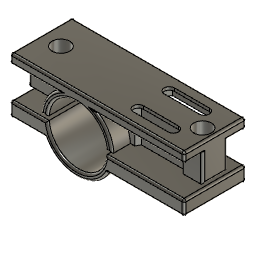
plate_holder (Autodesk Fusion 360 design; units mm, degrees)
Autodesk Fusion 360 part; units mm, degrees
sketch "Sketch1" plane through (0, 0, 0) normal (0, 1, 0) x (1, 0, 0)
  line L0 (17.1709, 1) -> (52.1709, 1)
  line L1 (52.1709, 1) -> (52.1709, 8)
  line L2 (52.1709, 8) -> (15.2263, 8)
  line L3 (17.1709, 1) -> (14.1647, 1)
  line L4 (0, 0) -> (0, 14.2)
  line L5 (-32.1709, 8) -> (-15.2263, 8)
  line L6 (-32.1709, 1) -> (-32.1709, 8)
  line L7 (-17.1709, 1) -> (-32.1709, 1)
  line L8 (-17.1709, 1) -> (-14.1647, 1)
  arc A0 (17.1709, 1) -> (-17.1709, 1) centre (0, 0) ccw
  arc A1 (14.1647, 1) -> (-14.1647, 1) centre (0, 0) ccw
  dimension "d1" = 28.4
  dimension "d3" = 1
  dimension "d4" = 7
  dimension "d5" = 35
  dimension "d6" = 34.4
  dimension "d64" = 15
  dimension "d65" = 7
  dimension "d66" = 1
  constraint coincident L4.start A0.centre
  constraint horizontal L0
  constraint perpendicular L0 L1
  constraint perpendicular L1 L2
  constraint parallel L0 L3
  constraint coincident L4.end A1
  constraint vertical L4
  constraint concentric A0 A1
  constraint coincident L5.end A0
  constraint parallel L0 L7
  constraint parallel L1 L6
  constraint parallel L2 L5
  constraint parallel L3 L8
  measures "d1" diameter of A1
  measures "d3" distance of L4.start L0
  measures "d4" distance of L0.end L1.end
  measures "d5" horizontal distance of L0.start L1.end
  measures "d6" diameter of A0
  measures "d64" distance of L6.start L7.start
  measures "d65" distance of L5.start L6.start
  measures "d66" distance of L7 L4.start
extrude "Extrude1" add sketch "Sketch1" along normal blind 30 makes body 1
sketch "Sketch2" plane through (0, 0, 0) normal (0, 1, 0) x (1, 0, 0)
  line L0 (17.1709, -1) -> (52.1709, -1)
  line L1 (52.1709, -1) -> (52.1709, -19)
  line L2 (52.1709, -19) -> (0, -19)
  line L3 (17.1709, -1) -> (14.1647, -1)
  line L4 (0, 0) -> (0, -19)
  line L5 (-32.1709, -19) -> (0, -19)
  line L6 (-32.1709, -1) -> (-32.1709, -19)
  line L7 (-17.1709, -1) -> (-32.1709, -1)
  line L8 (-17.1709, -1) -> (-14.1647, -1)
  arc A0 (-17.1709, -1) -> (17.1709, -1) centre (0, 0) ccw
  arc A1 (-14.1647, -1) -> (14.1647, -1) centre (0, 0) ccw
  line L9 (0, -14.2) -> (52.1709, -14.2)
  line L10 (0, -14.2) -> (-32.1709, -14.2)
  dimension "d9" = 28.4
  dimension "d10" = 34.4
  dimension "d11" = 1
  dimension "d12" = 35
  dimension "d14" = 18
  dimension "d67" = 18
  dimension "d68" = 15
  dimension "d69" = 1
  constraint coincident L4.start A0.centre
  constraint horizontal L0
  constraint perpendicular L0 L1
  constraint perpendicular L1 L2
  constraint vertical L4.start L2.end
  constraint parallel L0 L3
  constraint coincident L1 L9.end
  constraint perpendicular L1 L9
  constraint tangent A1 L9
  constraint coincident A1 L9.start
  constraint coincident L6 L10.end
  constraint parallel L1 L6
  constraint parallel L2 L5
  constraint parallel L9 L10
  constraint parallel L0 L8
  constraint coincident L9.start L10
  measures "d9" diameter of A1
  measures "d10" diameter of A0
  measures "d11" distance of L4.start L0
  measures "d12" distance of L0.start L0.end
  measures "d14" distance of L0 L2.end
  measures "d67" distance of L5 L7
  measures "d68" distance of L6.start L7.start
  measures "d69" distance of L4.start L7
extrude "Extrude2" add sketch "Sketch2" along normal up to surface (30 mm away) separate body contours L3 A0 A1 L9 | L1 L2 L4 A0 L9 | L4 A0 L9 | L8 A0 A1 L10 | L4 A0 L10 | L4 L5 L6 A0 L10 makes body 2
extrude "Extrude3" add sketch "Sketch2" along normal mid plane 12 from surface at 15 contours L0 L1 A0 L9 | L6 L7 A0 L10 bodies 2
sketch "Sketch3" plane through (0, 0, 19) normal (0, 0, 1) x (-1, 0, 0)
  line L0 (-52.1709, -30) -> (32.1709, -30)
  line L1 (32.1709, -30) -> (32.1709, 0)
  line L2 (32.1709, 0) -> (-52.1709, 0)
  line L3 (-52.1709, 0) -> (-52.1709, -30)
  line L4 (0, 0) -> (0, -30)
  circle A0 centre (-22.5, -7.5) radius 2.5
  line L5 (0, -15) -> (-52.1709, -15)
  circle A1 centre (-22.5, -22.5) radius 2.5
  circle A2 centre (-46.1709, -15) radius 2.075
  circle A3 centre (-46.1709, -15) radius 4.25
  circle A4 centre (22.5, -15) radius 4.25
  circle A5 centre (22.5, -15) radius 2.075
  line L6 (-22.5, -7.5) -> (-31, -7.5) construction
  line L7 (0, -15) -> (32.1709, -15) construction
  line L8 (-22.5, -7.5) -> (-52.1709, -7.5) construction
  circle A6 centre (-39.5, -7.5) radius 2.5
  circle A7 centre (-39.5, -22.5) radius 2.5
  line L9 (-22.5, -25) -> (-39.5, -25)
  line L10 (-22.5, -20) -> (-39.5, -20)
  line L11 (-22.5, -10) -> (-39.5, -10)
  line L12 (-22.5, -5) -> (-39.5, -5)
  dimension "d20" = 5
  dimension "d21" = 45
  dimension "d22" = 15
  dimension "d33" = 4.15
  dimension "d34" = 6
  dimension "d35" = 8.5
  dimension "d70" = 45
  dimension "d73" = 5
  dimension "d74" = 17
  dimension "d75" = 8.5
  dimension "d76" = 4.15
  constraint coincident L4.start origin
  constraint midpoint L4 L5.start
  constraint perpendicular L4 L5
  constraint symmetric A0 L5 A1
  constraint coincident L5 A2.centre
  constraint concentric A2 A3
  constraint coincident L3 L5.end
  constraint coincident A0.centre L6.start
  constraint horizontal L6
  constraint vertical L4
  constraint coincident L0 L4.end
  constraint midpoint L1 L7.end
  constraint coincident A4.centre L7
  constraint concentric A4 A5
  constraint perpendicular L3 L8
  constraint coincident L3 L8.end
  constraint coincident L8 A6.centre
  constraint symmetric L5 A6 A7
  constraint coincident A1 L9.start
  constraint coincident A7 L9.end
  constraint parallel L0 L9
  constraint coincident A1 L10.start
  constraint coincident A7 L10.end
  constraint parallel L9 L10
  constraint tangent A1 L9
  constraint tangent A7 L10
  constraint coincident A0 L11.start
  constraint coincident A6 L11.end
  constraint parallel L10 L11
  constraint coincident A0 L12.start
  constraint coincident A6 L12.end
  constraint parallel L8 L12
  constraint tangent A0 L11
  constraint tangent A6 L12
  measures "d20" diameter of A0
  measures "d33" diameter of A2
  measures "d34" distance of L3 A2.centre
  measures "d35" diameter of A3
  measures "d73" diameter of A6
  measures "d74" distance of A0.centre A6.centre
  measures "d75" diameter of A4
  measures "d76" diameter of A5
extrude "Extrude4" cut sketch "Sketch3" against normal up to surface (4.8 mm away) contours A0 | A0 A6 L11 L12 | A6 | A1 | A1 A7 L9 L10 | A7 bodies 2
sketch "Sketch4" plane through (0, 0, 14.2) normal (0, 0, -1) x (1, 0, 0)
  line L0 (41.5, -9) -> (52.1709, -9)
  line L1 (52.1709, -9) -> (52.1709, 0)
  line L2 (52.1709, 0) -> (9.7057, 0)
  line L3 (9.7057, 0) -> (9.7057, -9)
  line L4 (24.564, -3.925) -> (20.436, -3.925)
  line L5 (20.436, -3.925) -> (18.3719, -7.5)
  line L6 (18.3719, -7.5) -> (20.436, -11.075)
  line L7 (20.436, -11.075) -> (24.564, -11.075)
  line L8 (24.564, -11.075) -> (26.6281, -7.5)
  line L9 (26.6281, -7.5) -> (24.564, -3.925)
  line L10 (0, -15) -> (52.1709, -15) construction
  line L11 (52.1709, -9) -> (52.1709, -21)
  line L12 (0, -15) -> (0, 0) construction
  line L13 (20.436, -26.075) -> (18.3719, -22.5)
  line L14 (24.564, -26.075) -> (20.436, -26.075)
  line L15 (26.6281, -22.5) -> (24.564, -26.075)
  line L16 (24.564, -18.925) -> (26.6281, -22.5)
  line L17 (20.436, -18.925) -> (24.564, -18.925)
  line L18 (18.3719, -22.5) -> (20.436, -18.925)
  line L19 (-24.564, -3.925) -> (-20.436, -3.925)
  line L20 (-26.6281, -7.5) -> (-24.564, -3.925)
  circle A0 centre (-22.5, -7.5) radius 2.5
  line L21 (-18.3719, -7.5) -> (-20.436, -11.075)
  line L22 (-20.436, -3.925) -> (-18.3719, -7.5)
  line L23 (-20.436, -11.075) -> (-24.564, -11.075)
  line L24 (-24.564, -11.075) -> (-26.6281, -7.5)
  line L25 (-24.564, -18.925) -> (-26.6281, -22.5)
  line L26 (-20.436, -26.075) -> (-18.3719, -22.5)
  line L27 (-20.436, -18.925) -> (-24.564, -18.925)
  line L28 (-24.564, -26.075) -> (-20.436, -26.075)
  line L29 (-18.3719, -22.5) -> (-20.436, -18.925)
  line L30 (-26.6281, -22.5) -> (-24.564, -26.075)
  arc A1 (22.5, -5) -> (20.5, -9) centre (22.5, -7.5) ccw
  line L31 (9.7057, -9) -> (20.5, -9)
  arc A2 (41.5, -9) -> (39.5, -5) centre (39.5, -7.5) ccw
  line L32 (22.5, -5) -> (39.5, -5)
  line L33 (31, -9) -> (31, -6) construction
  line L34 (22.5, -7.5) -> (39.5, -7.5) construction
  line L35 (35.3719, -7.5) -> (37.436, -3.925)
  line L36 (37.436, -3.925) -> (41.564, -3.925)
  line L37 (41.564, -3.925) -> (43.6281, -7.5)
  line L38 (43.6281, -7.5) -> (41.564, -11.075)
  line L39 (41.564, -11.075) -> (37.436, -11.075)
  line L40 (37.436, -11.075) -> (35.3719, -7.5)
  line L41 (35.3719, -22.5) -> (37.436, -26.075)
  line L42 (37.436, -26.075) -> (41.564, -26.075)
  line L43 (41.564, -26.075) -> (43.6281, -22.5)
  line L44 (43.6281, -22.5) -> (41.564, -18.925)
  line L45 (41.564, -18.925) -> (37.436, -18.925)
  line L46 (37.436, -18.925) -> (35.3719, -22.5)
  line L47 (24.564, -3.925) -> (37.436, -3.925)
  line L48 (37.436, -11.075) -> (24.564, -11.075)
  line L49 (24.564, -18.925) -> (37.436, -18.925)
  line L50 (24.564, -26.075) -> (37.436, -26.075)
  point P0 (22.5, -7.5)
  point P1 (-22.5, -7.5)
  dimension "d25" = 7.15
  dimension "d26" = 7.5
  dimension "d77" = 3
  constraint coincident P0 A1.centre
  constraint parallel L2 L4
  constraint horizontal L10
  constraint coincident L10.end L11
  constraint vertical L12.end L10.start
  constraint coincident L12.end origin
  constraint symmetric L4.start L10 L14.start
  constraint symmetric L4.end L10 L13.start
  constraint symmetric L5.end L10 L13.end
  constraint symmetric L6.end L10 L17.start
  constraint symmetric L7.end L10 L16.start
  constraint symmetric L8.end L10 L15.start
  constraint symmetric L12 A0 A1
  constraint symmetric L4.start L12 L19.start
  constraint symmetric L4.end L12 L19.end
  constraint symmetric L5.end L12 L21.start
  constraint symmetric L6.end L12 L21.end
  constraint symmetric L7.end L12 L23.end
  constraint symmetric L8.end L12 L20.start
  constraint symmetric P0 L12 P1
  constraint symmetric L12 L13.start L26.start
  constraint symmetric L12 L13.end L26.end
  constraint symmetric L12 L14.start L28.start
  constraint symmetric L12 L15.start L25.end
  constraint symmetric L12 L16.start L25.start
  constraint symmetric L12 L17.start L27.start
  constraint perpendicular L32 L33
  constraint coincident A2.centre L34.end
  constraint midpoint L33 L34
  constraint symmetric L4.start L33 L35.end
  constraint symmetric L4.end L33 L36.end
  constraint symmetric L5.end L33 L37.end
  constraint symmetric L6.end L33 L38.end
  constraint symmetric L7.end L33 L39.end
  constraint symmetric L8.end L33 L35.start
  constraint symmetric L10 L35.start L41.start
  constraint symmetric L10 L35.end L41.end
  constraint symmetric L10 L36.end L42.end
  constraint symmetric L10 L37.end L43.end
  constraint symmetric L10 L38.end L44.end
  constraint symmetric L10 L39.end L45.end
  measures "d25" distance of L4 L7
  measures "d26" distance of P0 L10
  measures "d77" distance of L33.start L33.end
extrude "Extrude5" cut sketch "Sketch4" against normal up to surface (3.3 mm away) contours L0 A2 L32 L35 L36 L37 L38 | L0 A2 L32 L35 L38 L39 L40 | L8 L9 L32 L35 L40 L48 | L9 L32 L35 L47 | L4 L5 L6 L9 A1 L31 L32 | L6 L7 L8 L9 A1 L31 L32 | L13 L14 L15 L16 L17 L18 | L15 L16 L41 L46 L49 L50 | L41 L42 L43 L44 L45 L46 bodies 2
sketch "Sketch5" plane through (0, 0, 1) normal (0, 0, -1) x (1, 0, 0)
  line L0 (-17.1709, -30) -> (-14.1647, -30)
  line L1 (-14.1647, -30) -> (-14.1647, 0)
  line L2 (-14.1647, 0) -> (-17.1709, 0)
  line L3 (-17.1709, 0) -> (-17.1709, -9)
  line L4 (-17.1709, -9) -> (-32.1709, -9)
  line L5 (-32.1709, -9) -> (-32.1709, -21)
  line L6 (-32.1709, -21) -> (-17.1709, -21)
  line L7 (-17.1709, -21) -> (-17.1709, -30)
  line L8 (20.436, -3.925) -> (41.564, -3.925)
  line L9 (31, -3.925) -> (31, -9) construction
  line L10 (0, 0) -> (0, -30) construction
  line L11 (-14.1647, -30) -> (14.1647, -30)
  line L12 (0, -15) -> (52.1709, -15)
  line L13 (52.1709, -9) -> (52.1709, -21)
  point P0 (31, -3.925)
  point P1 (0, -15)
  constraint midpoint P0 L8
  constraint coincident P0 L9.start
  constraint perpendicular L8 L9
  constraint coincident L10.start origin
  constraint vertical L10
  constraint coincident L10.end L11
  constraint coincident L10 P1
  constraint midpoint L10 P1
  constraint coincident P1 L12.start
  constraint perpendicular L10 L12
  constraint coincident L12.end L13
sketch "Sketch6" plane through (0, 0, 19) normal (0, 0, 1) x (-1, 0, 0)
  line L0 (-52.1709, -30) -> (32.1709, -30)
  line L1 (32.1709, -30) -> (32.1709, 0)
  line L2 (32.1709, 0) -> (-52.1709, 0)
  line L3 (-52.1709, 0) -> (-52.1709, -30)
  line L4 (-22.5, -25) -> (-39.5, -25)
  arc A0 (-39.5, -20) -> (-39.5, -25) centre (-39.5, -22.5) ccw
  line L5 (-39.5, -20) -> (-22.5, -20)
  arc A1 (-22.5, -25) -> (-22.5, -20) centre (-22.5, -22.5) ccw
  line L6 (-22.5, -10) -> (-39.5, -10)
  arc A2 (-39.5, -5) -> (-39.5, -10) centre (-39.5, -7.5) ccw
  line L7 (-39.5, -5) -> (-22.5, -5)
  arc A3 (-22.5, -10) -> (-22.5, -5) centre (-22.5, -7.5) ccw
extrude "Extrude7" cut sketch "Sketch3" against normal up to surface (18 mm away) contours L5 A2 | L5 A2 | A5 bodies 2
extrude "Extrude8" cut sketch "Sketch3" against normal up to surface (16.5 mm away) contours L5 A2 A3 | L5 A2 A3 | A4 bodies 2
sketch "Sketch7" plane through (0, 0, -8) normal (0, 0, -1) x (1, 0, 0)
  line L0 (52.1709, 0) -> (15.2263, 0)
  line L1 (15.2263, 0) -> (15.2263, -30)
  line L2 (15.2263, -30) -> (52.1709, -30)
  line L3 (52.1709, -30) -> (52.1709, 0)
  line L4 (0, 0) -> (0, -30) construction
  line L5 (-15.2263, -30) -> (15.2263, -30)
  line L6 (0, -15) -> (52.1709, -15) construction
  circle A0 centre (46.1709, -15) radius 2.075
  line L7 (44.1069, -18.575) -> (48.2349, -18.575)
  line L8 (48.2349, -18.575) -> (50.299, -15)
  line L9 (50.299, -15) -> (48.2349, -11.425)
  line L10 (48.2349, -11.425) -> (44.1069, -11.425)
  line L11 (44.1069, -11.425) -> (42.0429, -15)
  line L12 (42.0429, -15) -> (44.1069, -18.575)
  circle A1 centre (-22.5, -15) radius 2.075
  circle A2 centre (-22.5, -15) radius 2.075
  line L13 (-18.3719, -15) -> (-20.436, -11.425)
  line L14 (-20.436, -11.425) -> (-24.564, -11.425)
  line L15 (-24.564, -11.425) -> (-26.6281, -15)
  line L16 (-26.6281, -15) -> (-24.564, -18.575)
  line L17 (-24.564, -18.575) -> (-20.436, -18.575)
  line L18 (-20.436, -18.575) -> (-18.3719, -15)
  point P0 (0, -15)
  point P1 (46.1709, -15)
  point P2 (-22.5, -15)
  dimension "d40" = 6
  dimension "d41" = 4.15
  dimension "d42" = 7.15
  dimension "d71" = 7.15
  dimension "d72" = 4.15
  constraint coincident L4.start origin
  constraint parallel L3 L4
  constraint coincident L4.end L5
  constraint coincident L4 P0
  constraint midpoint L4 P0
  constraint coincident P0 L6.start
  constraint perpendicular L1 L6
  constraint coincident L3 L6.end
  constraint coincident L6 P1
  constraint coincident P1 A0.centre
  constraint parallel L6 L7
  constraint concentric A1 A2
  constraint coincident P2 A1.centre
  constraint parallel L7 L17
  measures "d40" distance of L3 P1
  measures "d41" diameter of A0
  measures "d42" distance of L7 L10
  measures "d71" distance of L14 L17
  measures "d72" diameter of A1
extrude "Extrude9" cut sketch "Sketch7" against normal up to surface (7 mm away) contours A0 | A1 A2 bodies 1
extrude "Extrude10" cut sketch "Sketch7" against normal up to surface (5.5 mm away) contours L7 L8 L9 L10 L11 L12 | L13 L14 L15 L16 L17 L18 bodies 1
fillet "Fillet2" radius 1 8 faces at (27.1873, 30, -3.3333) (27.1873, 0, -3.3333) (-32.1709, 10, -3.3333) (52.1709, 10, -3.3333) (9.9019, 30, 17.4) (9.9019, 0, 17.4) (-32.1709, 17, 5.4) (52.1709, 13, 5.4) on bodies 1 2
sketch "Sketch10" plane through (0, 0, 17.5) normal (0, 0, -1) x (1, 0, 0)
  line L0 (39.5, -10) -> (22.5, -10)
  arc A0 (22.5, -5) -> (22.5, -10) centre (22.5, -7.5) ccw
  line L1 (22.5, -5) -> (39.5, -5)
  arc A1 (39.5, -10) -> (39.5, -5) centre (39.5, -7.5) ccw
  line L2 (20.436, -3.925) -> (18.3719, -7.5)
  line L3 (18.3719, -7.5) -> (20.436, -11.075)
  line L4 (20.436, -11.075) -> (41.564, -11.075)
  line L5 (41.564, -11.075) -> (43.6281, -7.5)
  line L6 (43.6281, -7.5) -> (41.564, -3.925)
  line L7 (41.564, -3.925) -> (20.436, -3.925)
  line L8 (20.436, -3.925) -> (18.3719, -7.5)
  line L9 (18.3719, -7.5) -> (20.436, -11.075)
  line L10 (20.436, -11.075) -> (41.564, -11.075)
  line L11 (41.564, -11.075) -> (43.6281, -7.5)
  line L12 (43.6281, -7.5) -> (41.564, -3.925)
  line L13 (41.564, -3.925) -> (20.436, -3.925)
  line L14 (0, -15) -> (52.1709, -15)
  line L15 (20.436, -18.925) -> (41.564, -18.925)
  line L16 (41.564, -18.925) -> (43.6281, -22.5)
  line L17 (43.6281, -22.5) -> (41.564, -26.075)
  line L18 (41.564, -26.075) -> (20.436, -26.075)
  line L19 (20.436, -26.075) -> (18.3719, -22.5)
  line L20 (18.3719, -22.5) -> (20.436, -18.925)
  dimension "d87" = 0
  constraint symmetric L2.start L14 L18.end
  constraint symmetric L2.end L14 L19.end
  constraint symmetric L3.end L14 L15.start
  constraint symmetric L4.end L14 L15.end
  constraint symmetric L5.end L14 L16.end
  constraint symmetric L6.end L14 L17.end
extrude "Extrude15" cut sketch "Sketch10" along normal up to surface (16.5 mm away) contours L0 A0 L1 A1 | L2 L3 L4 L5 L6 L7 L8 L9 L10 L11 L12 L13 | L15 L16 L17 L18 L19 L20 bodies 2
equation "d6 = 28.4 mm + 6 mm"
equation "d10 = 28.4 mm + 6 mm"
